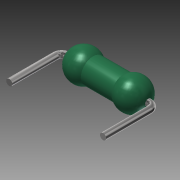
# Autodesk Inventor part: Resistor
Saved by Autodesk Inventor 2014 SP1 (Build 180222100, 222)
## iProperties
Created: 2016-03-19
Part Number: Resistor
Material: Generic
Document SubType Name: Modeling
Designer: Tyler
Density: 1 g/cm^3
Appearance: Smooth - Dark Sea Green
Author: Tyler
Autodesk Inventor part; units mm, degrees
ref_plane "YZ Plane" through (0, 0, 0) normal (1, 0, 0) x (0, 1, 0)
ref_plane "XZ Plane" through (0, 0, 0) normal (0, 1, 0) x (-1, 0, 0)
ref_plane "XY Plane" through (0, 0, 0) normal (0, 0, 1) x (1, 0, 0)
sketch "Sketch1" plane through (0, 0, 0) normal (0, 0, 1) x (1, 0, 0)
  arc A0 (-1.25, 1) -> (-3.25, 0) centre (-2, 0) ccw
  line L0 (0, 1) -> (-1.25, 1)
  line L1 (0, 0) -> (-3.25, 0)
  line L2 (0, 1) -> (0, 0) construction
  arc A1 (3.25, 0) -> (1.25, 1) centre (2, 0) ccw
  line L3 (0, 1) -> (1.25, 1)
  line L4 (0, 0) -> (3.25, 0)
  dimension "d0" = 2.5
  dimension "d2" = 1
  dimension "d5" = 0
  dimension "d6" = 0
  dimension "d11" = 3.25
  constraints: 10 end point, 4 point on circle, 3 symmetric about line, 2 centre point, 1 parallel, 1 perpendicular, 1 other
  measures "d0" diameter of A0
  measures "d2" distance from line of L1.start L0
  measures "d5" vertical distance of L1.start A0.centre
  measures "d6" vertical distance of L1.start L1.end
  measures "d11" distance of L1.start L1.end
revolve "Revolution1" add sketch "Sketch1" angle 360 about axis through (0, 0, 0) along (1, 0, 0)
sketch "Sketch2" plane through (0, 0, 0) normal (0, 0, 1) x (1, 0, 0)
  line L0 (-3.31, 0) -> (3.31, 0)
  line L1 (3.81, -0.5) -> (3.81, -4.25)
  line L2 (-3.81, -0.5) -> (-3.81, -4.25)
  arc A0 (-3.31, 0) -> (-3.81, -0.5) centre (-3.31, -0.5) ccw
  arc A1 (3.81, -0.5) -> (3.31, 0) centre (3.31, -0.5) ccw
  point P0 (0, 0)
  dimension "d8" = 4.25
  dimension "d9" = 7.62
  dimension "d10" = 3.81
  dimension "d12" = 0.5
  dimension "d13" = 0
  dimension "d14" = 4.25
  constraints: 6 end point, 4 point on circle, 4 tangent, 2 centre point, 1 equal radius, 1 horizontal, 1 parallel, 1 perpendicular
  measures "d8" distance from line of L2.end L0
  measures "d9" distance between parallel lines of L1 L2
  measures "d10" distance from line of point (0, 0) L1
  measures "d12" radius of A0
  measures "d13" distance from line of L0 point (0, 0)
  measures "d14" distance from line of L1.end L0
sketch "Sketch3" plane through (0, 0, 0) normal (1, 0, 0) x (0, 1, 0)
  circle A0 centre (0, 0) radius 0.25
  dimension "d15" = 0.5
  constraints: 1 centre point, 1 coincident
  measures "d15" diameter of A0
sweep "Sweep1" add profiles "Sketch3" path "Sketch2"
equation "\"d10\" = 0.5 * d9"
equation "\"d14\" = d8"
body "Solid1"
